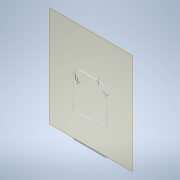
# Autodesk Inventor part: end body
Saved by Autodesk Inventor 2021 (Build 250183000, 183)
## iProperties
Created: 2021-11-16
Part Number: end body
Material: Generic
Document SubType Name: Modeling
Designer: jston
Density: 1 g/cm^3
Appearance: Default
Author: jston
Autodesk Inventor part; units mm, degrees
ref_plane "YZ Plane" through (0, 0, 0) normal (1, 0, 0) x (0, 1, 0)
ref_plane "XZ Plane" through (0, 0, 0) normal (0, 1, 0) x (-1, 0, 0)
ref_plane "XY Plane" through (0, 0, 0) normal (0, 0, 1) x (1, 0, 0)
ref_plane "Work Plane1" through (-878.5434, 221.5358, -1189.8607) normal (0, 0, 1) x (1, 0, 0)
sketch "Sketch2" plane through (-878.5434, 221.5358, -1189.8607) normal (0, 0, 1) x (1, 0, 0)
  line L0 (431.8, -127) -> (431.8, -304.8)
  line L1 (431.8, -304.8) -> (431.8, -393.7)
  line L2 (431.8, -393.7) -> (431.8, -635)
  line L3 (431.8, -635) -> (-127, -635)
  line L4 (-127, -635) -> (-127, -304.8)
  line L5 (-127, -304.8) -> (-127, -127)
  line L6 (304.8, 0) -> (0, 0)
  arc A0 (0, 12.7) -> (-139.7, -127) centre (0, -127) ccw construction
  line L7 (0, 12.7) -> (0, 11.049)
  arc A1 (0, 11.049) -> (-138.049, -127) centre (0, -127) ccw construction
  line L8 (-138.049, -127) -> (-139.7, -127)
  arc A2 (0, -12.7) -> (-114.3, -127) centre (0, -127) ccw construction
  line L9 (-114.3, -127) -> (-115.951, -127)
  arc A3 (0, -11.049) -> (-115.951, -127) centre (0, -127) ccw construction
  line L10 (0, -11.049) -> (0, -12.7)
  arc A4 (444.5, -127) -> (304.8, 12.7) centre (304.8, -127) ccw construction
  line L11 (444.5, -127) -> (442.849, -127)
  arc A5 (442.849, -127) -> (304.8, 11.049) centre (304.8, -127) ccw construction
  line L12 (304.8, 11.049) -> (304.8, 12.7)
  arc A6 (419.1, -127) -> (304.8, -12.7) centre (304.8, -127) ccw construction
  line L13 (304.8, -12.7) -> (304.8, -11.049)
  arc A7 (420.751, -127) -> (304.8, -11.049) centre (304.8, -127) ccw construction
  line L14 (420.751, -127) -> (419.1, -127)
  line L15 (0, -127) -> (179.6051, -127) construction
  line L16 (0, -127) -> (-80.8223, -46.1777) construction
  line L17 (-81.9897, -45.0103) -> (-97.6154, -29.3846)
  line L18 (-98.7828, -28.2172) -> (-127, 0)
  arc A8 (0, 0) -> (-127, -127) centre (0, -127) ccw
  line L19 (152.4, 0) -> (152.4, -147.1377) construction
  arc A9 (431.8, -127) -> (304.8, 0) centre (304.8, -127) ccw
  line L20 (-152.4, -127) -> (-152.4, -304.8)
  line L21 (-152.4, -304.8) -> (-152.4, -635)
  line L22 (457.2, -635) -> (457.2, -393.7)
  line L23 (457.2, -393.7) -> (457.2, -304.8)
  line L24 (457.2, -304.8) -> (457.2, -127)
  arc A10 (457.2, -127) -> (304.8, 25.4) centre (304.8, -127) ccw
  line L25 (304.8, 25.4) -> (0, 25.4)
  arc A11 (0, 25.4) -> (-152.4, -127) centre (0, -127) ccw
  line L26 (-153.9875, -304.8) -> (-153.9875, -127)
  arc A12 (0, 26.9875) -> (-153.9875, -127) centre (0, -127) ccw
  line L27 (0, 26.9875) -> (304.8, 26.9875)
  arc A13 (458.7875, -127) -> (304.8, 26.9875) centre (304.8, -127) ccw
  line L28 (458.7875, -127) -> (458.7875, -304.8)
  line L29 (458.7875, -304.8) -> (458.7875, -393.7)
  line L30 (458.7875, -393.7) -> (458.7875, -635)
  line L31 (-153.9875, -635) -> (-153.9875, -304.8)
  line L32 (431.8, -635) -> (458.7875, -635)
  line L33 (-127, -635) -> (-153.9875, -635)
  point P0 (878.5434, -221.5358)
  point P1 (-89.8026, -37.1974)
  point P2 (-107.7631, -19.2369)
  point P3 (-108.8856, -18.1144)
  dimension "d1" = 25.4
  dimension "d2" = 1.5875
  constraints: 68 end point, 33 point on circle, 14 centre point, 9 collinear, 6 horizontal, 6 vertical, 3 perpendicular, 3 point on line, 2 midpoint, 1 symmetric about line, 51 other
  measures "d1" distance between parallel lines of L5 L20
  measures "d2" distance between parallel lines of L20 L26
extrude "Extrusion2" add sketch "Sketch2" along normal blind 25.4 contours L22 L23 L24 A10 L25 A11 L18 A12 L27 A13 L28 L29 L30 L32 | L33 L31 L26 A12 L18 A11 L20 L21
body "Solid2"
